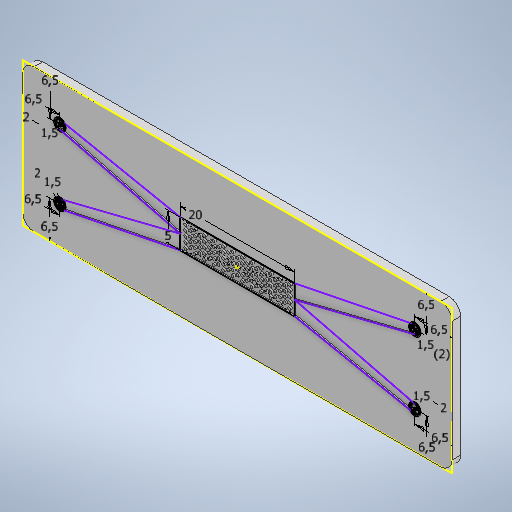
# Autodesk Inventor part: LAB1
Saved by Autodesk Inventor 2025.1 (Build 291241020, 241B)
## iProperties
Created: 2024-09-21
Part Number: LAB1
Material: Generic
Document SubType Name: Modeling
Designer: tomky
Density: 1 g/cm^3
Appearance: Default
Author: tomky
Autodesk Inventor part; units mm, degrees
ref_plane "YZ Plane" through (0, 0, 0) normal (1, 0, 0) x (0, 1, 0)
ref_plane "XZ Plane" through (0, 0, 0) normal (0, 1, 0) x (-1, 0, 0)
ref_plane "XY Plane" through (0, 0, 0) normal (0, 0, 1) x (1, 0, 0)
sketch "Sketch1" plane through (0, 0, 0) normal (0, 0, 1) x (1, 0, 0)
  line L0 (-37.5, 12.5) -> (37.5, 12.5)
  line L1 (37.5, 12.5) -> (37.5, -12.5)
  line L2 (37.5, -12.5) -> (-37.5, -12.5)
  line L3 (-37.5, -12.5) -> (-37.5, 12.5)
  line L4 (-37.5, 12.5) -> (37.5, -12.5) construction
  line L5 (37.5, 12.5) -> (-37.5, -12.5) construction
  point P0 (0, 0)
  dimension "d0" = 75
  dimension "d1" = 25
  constraints: 12 end point, 2 midpoint, 2 parallel, 1 horizontal, 1 perpendicular
  measures "d0" distance of L0.start L0.end
  measures "d1" distance of L0.end L1.end
extrude "Extrusion1" add sketch "Sketch1" along normal blind 1.5
sketch "Sketch2" plane through (0, 0, 1.5) normal (0, 0, 1) x (1, 0, 0)
  line L0 (-37.5, -12.5) -> (37.5, -12.5) projected
  circle A0 centre (31, -6) radius 1
  line L1 (37.5, -12.5) -> (37.5, 12.5) projected
  circle A1 centre (31, 6) radius 1
  line L2 (37.5, 12.5) -> (-37.5, 12.5) projected
  circle A2 centre (-31, 6) radius 1
  line L3 (-37.5, 12.5) -> (-37.5, -12.5) projected
  circle A3 centre (-31, -6) radius 1
  circle A4 centre (-31, 6) radius 0.75
  circle A5 centre (-31, -6) radius 0.75
  circle A6 centre (31, -6) radius 0.75
  circle A7 centre (31, 6) radius 0.75
  line L4 (10, -2.5) -> (-10, -2.5)
  line L5 (-10, -2.5) -> (-10, 2.5)
  line L6 (-10, 2.5) -> (10, 2.5)
  line L7 (10, 2.5) -> (10, -2.5)
  line L8 (10, -2.5) -> (-10, 2.5) construction
  line L9 (-10, -2.5) -> (10, 2.5) construction
  line L10 (31, 6.75) -> (10, 2.5)
  line L11 (31, 5.25) -> (10, 0)
  line L12 (31, -5.25) -> (10, 0)
  line L13 (31, -6.75) -> (10, -2.5)
  line L14 (-31, -5.25) -> (-10, 0)
  line L15 (-31, -6.75) -> (-10, -2.5)
  line L16 (-31, 5.25) -> (-10, 0)
  line L17 (-31, 6.75) -> (-10, 2.5)
  point P0 (0, 0)
  point P1 (30.1897, 6.586)
  point P2 (-30.1897, 6.586)
  point P3 (-30.511, 5.1277)
  point P4 (-30.511, -5.1277)
  point P5 (-30.1897, -6.586)
  point P6 (30.1897, -6.586)
  point P7 (30.511, -5.1277)
  point P8 (30.511, 5.1277)
  dimension "d6" = 2
  dimension "d7" = 6.5
  dimension "d8" = 6.5
  dimension "d9" = 2
  dimension "d10" = 6.5
  dimension "d11" = 6.5
  dimension "d12" = 2
  dimension "d13" = 6.5
  dimension "d14" = 6.5
  dimension "d15" = 2
  dimension "d16" = 6.5
  dimension "d17" = 6.5
  dimension "d18" = 1.5
  dimension "d19" = 1.5
  dimension "d20" = 1.5
  dimension "d21" = 1.5
  dimension "d22" = 20
  dimension "d23" = 5
  constraints: 28 end point, 8 centre point, 8 point on circle, 4 coincident, 4 midpoint, 3 parallel, 1 equal radius, 1 horizontal, 1 perpendicular
  measures "d6" diameter of A0
  measures "d7" distance from line of L0 A0.centre
  measures "d8" distance from line of L1 A0.centre
  measures "d9" diameter of A1
  measures "d10" distance from line of L1 A1.centre
  measures "d11" distance from line of L2 A1.centre
  measures "d12" diameter of A2
  measures "d13" distance from line of L2 A2.centre
  measures "d14" distance from line of L3 A2.centre
  measures "d15" diameter of A3
  measures "d16" distance from line of L3 A3.centre
  measures "d17" distance from line of L0 A3.centre
  measures "d18" diameter of A4
  measures "d19" diameter of A5
  measures "d20" diameter of A6
  measures "d21" diameter of A7
  measures "d22" distance of L5.end L6.end
  measures "d23" distance of L4.end L5.end
extrude "Extrusion2" add sketch "Sketch2" against normal blind 6.5 contours A0 L13 A6 L12 | L12 A6 L13 A0 | A6 L13 | L13 A6 | L11 A7 L10 A1 | A1 L10 A7 L11 | A7 L10 | L15 A5 L14 A3 | A3 L14 A5 L15 | L17 A4 L16 A2 | A2 L16 A4 L17 | A7 L10 | L15 A5 | A5 L15 | L17 A4 | A4 L17
extrude "Extrusion3" cut sketch "Sketch2" against normal through all contours A6 L13 | L13 A6 | A7 L10 | A7 L10 | L15 A5 | A5 L15 | L17 A4 | A4 L17
fillet "Fillet1" radius 0.5 4 edges at (30, 6, 0) (30, -6, 0) (-32, -6, 0) (-32, 6, 0)
extrude "Extrusion4" cut sketch "Sketch2" against normal blind 0.3 contours A0 L13 A6 L12 | L12 A6 L13 A0 | A0 L13 L7 L12 | A6 L13 | L7 L4 L5 L6 | L7 L10 A1 L11 | L13 A6 | L11 A7 L10 A1 | A1 L10 A7 L11 | L15 A3 L14 L5 | L5 L16 A2 L17 | A7 L10 | L15 A5 L14 A3 | A3 L14 A5 L15 | L17 A4 L16 A2 | A2 L16 A4 L17 | A7 L10 | L15 A5 | A5 L15 | L17 A4 | A4 L17
sketch "Sketch3" plane through (0, 0, 1.2) normal (0, 0, 1) x (1, 0, 0)
  line L0 (10, -2.5) -> (-10, -2.5) construction
  line L1 (-10, 2.5) -> (10, 2.5) construction
  line L2 (0, 2.5) -> (0, -2.5) construction
  line L3 (-30.511, -5.1277) -> (-10, 0) projected
  line L4 (30.511, 5.1277) -> (10, 0) projected
  line L5 (-10, 0) -> (10, 0) construction
  circle A0 centre (0, 0.4) radius 0.25
  circle A1 centre (0, 1.3) radius 0.25
  circle A2 centre (0.8062, 0) radius 0.25
  circle A3 centre (0.8062, 0.9) radius 0.25
  circle A4 centre (0.8062, 1.8) radius 0.25
  circle A5 centre (2.4562, 0) radius 0.25
  circle A6 centre (2.4562, 0.9) radius 0.25
  circle A7 centre (2.4562, 1.8) radius 0.25
  circle A8 centre (1.65, 0.4) radius 0.25
  circle A9 centre (1.65, 1.3) radius 0.25
  circle A10 centre (4.1062, 0) radius 0.25
  circle A11 centre (4.1062, 0.9) radius 0.25
  circle A12 centre (4.1062, 1.8) radius 0.25
  circle A13 centre (3.3, 0.4) radius 0.25
  circle A14 centre (3.3, 1.3) radius 0.25
  circle A15 centre (5.7562, 0) radius 0.25
  circle A16 centre (5.7562, 0.9) radius 0.25
  circle A17 centre (5.7562, 1.8) radius 0.25
  circle A18 centre (4.95, 0.4) radius 0.25
  circle A19 centre (4.95, 1.3) radius 0.25
  circle A20 centre (7.4062, 0) radius 0.25
  circle A21 centre (7.4062, 0.9) radius 0.25
  circle A22 centre (7.4062, 1.8) radius 0.25
  circle A23 centre (6.6, 0.4) radius 0.25
  circle A24 centre (6.6, 1.3) radius 0.25
  circle A25 centre (9.0562, 0) radius 0.25
  circle A26 centre (9.0562, 0.9) radius 0.25
  circle A27 centre (9.0562, 1.8) radius 0.25
  circle A28 centre (8.25, 0.4) radius 0.25
  circle A29 centre (8.25, 1.3) radius 0.25
  circle A30 centre (10.7062, 0) radius 0.25
  circle A31 centre (10.7062, 0.9) radius 0.25
  circle A32 centre (10.7062, 1.8) radius 0.25
  circle A33 centre (9.9, 0.4) radius 0.25
  circle A34 centre (9.9, 1.3) radius 0.25
  circle A35 centre (-1.65, 1.3) radius 0.25
  circle A36 centre (-1.65, 0.4) radius 0.25
  circle A37 centre (-0.8438, 0) radius 0.25
  circle A38 centre (-0.8438, 0.9) radius 0.25
  circle A39 centre (-0.8438, 1.8) radius 0.25
  circle A40 centre (-3.3, 1.3) radius 0.25
  circle A41 centre (-3.3, 0.4) radius 0.25
  circle A42 centre (-2.4938, 0) radius 0.25
  circle A43 centre (-2.4938, 0.9) radius 0.25
  circle A44 centre (-2.4938, 1.8) radius 0.25
  circle A45 centre (-4.95, 1.3) radius 0.25
  circle A46 centre (-4.95, 0.4) radius 0.25
  circle A47 centre (-4.1438, 0) radius 0.25
  circle A48 centre (-4.1438, 0.9) radius 0.25
  circle A49 centre (-4.1438, 1.8) radius 0.25
  circle A50 centre (-6.6, 1.3) radius 0.25
  circle A51 centre (-6.6, 0.4) radius 0.25
  circle A52 centre (-5.7938, 0) radius 0.25
  circle A53 centre (-5.7938, 0.9) radius 0.25
  circle A54 centre (-5.7938, 1.8) radius 0.25
  circle A55 centre (-8.25, 1.3) radius 0.25
  circle A56 centre (-8.25, 0.4) radius 0.25
  circle A57 centre (-7.4438, 0) radius 0.25
  circle A58 centre (-7.4438, 0.9) radius 0.25
  circle A59 centre (-7.4438, 1.8) radius 0.25
  circle A60 centre (-9.9, 1.3) radius 0.25
  circle A61 centre (-9.9, 0.4) radius 0.25
  circle A62 centre (-9.0938, 0) radius 0.25
  circle A63 centre (-9.0938, 0.9) radius 0.25
  circle A64 centre (-9.0938, 1.8) radius 0.25
  line L6 (-10, -2.5) -> (10, -2.5) construction
  circle A65 centre (0, -0.4) radius 0.25
  circle A66 centre (0, -1.3) radius 0.25
  circle A67 centre (0.8062, 0) radius 0.25
  circle A68 centre (0.8062, -0.9) radius 0.25
  circle A69 centre (0.8062, -1.8) radius 0.25
  circle A70 centre (2.4562, 0) radius 0.25
  circle A71 centre (2.4562, -0.9) radius 0.25
  circle A72 centre (2.4562, -1.8) radius 0.25
  circle A73 centre (1.65, -0.4) radius 0.25
  circle A74 centre (1.65, -1.3) radius 0.25
  circle A75 centre (4.1062, 0) radius 0.25
  circle A76 centre (4.1062, -0.9) radius 0.25
  circle A77 centre (4.1062, -1.8) radius 0.25
  circle A78 centre (3.3, -0.4) radius 0.25
  circle A79 centre (3.3, -1.3) radius 0.25
  circle A80 centre (5.7562, 0) radius 0.25
  circle A81 centre (5.7562, -0.9) radius 0.25
  circle A82 centre (5.7562, -1.8) radius 0.25
  circle A83 centre (4.95, -0.4) radius 0.25
  circle A84 centre (4.95, -1.3) radius 0.25
  circle A85 centre (7.4062, 0) radius 0.25
  circle A86 centre (7.4062, -0.9) radius 0.25
  circle A87 centre (7.4062, -1.8) radius 0.25
  circle A88 centre (6.6, -0.4) radius 0.25
  circle A89 centre (6.6, -1.3) radius 0.25
  circle A90 centre (9.0562, 0) radius 0.25
  circle A91 centre (9.0562, -0.9) radius 0.25
  circle A92 centre (9.0562, -1.8) radius 0.25
  circle A93 centre (8.25, -0.4) radius 0.25
  circle A94 centre (8.25, -1.3) radius 0.25
  circle A95 centre (9.9, -0.4) radius 0.25
  circle A96 centre (9.9, -1.3) radius 0.25
  circle A97 centre (-1.65, -1.3) radius 0.25
  circle A98 centre (-1.65, -0.4) radius 0.25
  circle A99 centre (-0.8438, 0) radius 0.25
  circle A100 centre (-0.8438, -0.9) radius 0.25
  circle A101 centre (-0.8438, -1.8) radius 0.25
  circle A102 centre (-3.3, -1.3) radius 0.25
  circle A103 centre (-3.3, -0.4) radius 0.25
  circle A104 centre (-2.4938, 0) radius 0.25
  circle A105 centre (-2.4938, -0.9) radius 0.25
  circle A106 centre (-2.4938, -1.8) radius 0.25
  circle A107 centre (-4.95, -1.3) radius 0.25
  circle A108 centre (-4.95, -0.4) radius 0.25
  circle A109 centre (-4.1438, 0) radius 0.25
  circle A110 centre (-4.1438, -0.9) radius 0.25
  circle A111 centre (-4.1438, -1.8) radius 0.25
  circle A112 centre (-6.6, -1.3) radius 0.25
  circle A113 centre (-6.6, -0.4) radius 0.25
  circle A114 centre (-5.7938, 0) radius 0.25
  circle A115 centre (-5.7938, -0.9) radius 0.25
  circle A116 centre (-5.7938, -1.8) radius 0.25
  circle A117 centre (-8.25, -1.3) radius 0.25
  circle A118 centre (-8.25, -0.4) radius 0.25
  circle A119 centre (-7.4438, 0) radius 0.25
  circle A120 centre (-7.4438, -0.9) radius 0.25
  circle A121 centre (-7.4438, -1.8) radius 0.25
  circle A122 centre (-9.9, -1.3) radius 0.25
  circle A123 centre (-9.9, -0.4) radius 0.25
  circle A124 centre (-9.0938, 0) radius 0.25
  circle A125 centre (-9.0938, -0.9) radius 0.25
  circle A126 centre (-9.0938, -1.8) radius 0.25
  point P0 (0, 0)
  point P1 (0, 0)
  point P2 (1.65, 0)
  point P3 (3.3, 0)
  point P4 (4.95, 0)
  point P5 (6.6, 0)
  point P6 (8.25, 0)
  point P7 (9.9, 0)
  point P8 (-1.65, 0)
  point P9 (-1.65, 0)
  point P10 (-3.3, 0)
  point P11 (-3.3, 0)
  point P12 (-4.95, 0)
  point P13 (-4.95, 0)
  point P14 (-6.6, 0)
  point P15 (-6.6, 0)
  point P16 (-8.25, 0)
  point P17 (-8.25, 0)
  point P18 (-9.9, 0)
  point P19 (-9.9, 0)
  dimension "d31" = 0.5
  dimension "d32" = 0
  dimension "d33" = 0.4
  dimension "d34" = 0.5
  dimension "d35" = 0.4
  dimension "d36" = 0.5
  dimension "d37" = 0.4
  dimension "d38" = 0.5
  dimension "d41" = 0.4
  dimension "d42" = 0.5
  dimension "d43" = 0.4
  dimension "d46" = 1.65
  dimension "d53" = 1.65
  constraints: 127 centre point, 50 symmetric about line, 6 end point, 3 midpoint, 2 horizontal, 2 point on line, 2 vertical alignment, 1 perpendicular, 200 other
  measures "d31" diameter of A0
  measures "d32" distance from line of L2 A0.centre
  measures "d33" distance of point (0, 0) A0.centre
  measures "d34" diameter of A1
  measures "d36" diameter of A2
  measures "d37" vertical distance between centres of A0 A2
  measures "d38" diameter of A3
  measures "d42" diameter of A4
  measures "d46" distance of A0.centre A8.centre
  measures "d53" distance of A1.centre A35.centre
extrude "Extrusion5" add sketch "Sketch3" along normal blind 0.3 contours A0 | A1 | A2 | A3 | A4 | A5 | A6 | A7 | A8 | A9 | A10 | A11 | A12 | A13 | A14 | A15 | A16 | A17 | A18 | A19 | A20 | A21 | A22 | A23 | A24 | A25 | A26 | A27 | A28 | A29 | A35 | A36 | A37 | A38 | A39 | A40 | A41 | A42 | A43 | A44 | A45 | A46 | A47 | A48 | A49 | A50 | A51 | A52 | A53 | A54 | A55 | A56 | A57 | A58 | A59 | A62 | A63 | A64 | A65 | A66 | A68 | A69 | A71 | A72 | A73 | A74 | A76 | A77 | A78 | A79 | A81 | A82 | A83 | A84 | A86 | A87 | A88 | A89 | A91 | A92 | A93 | A94 | A97 | A98 | A100 | A101 | A102 | A103 | A105 | A106 | A107 | A108 | A110 | A111 | A112 | A113 | A115 | A116 | A117 | A118 | A120 | A121 | A125 | A126
sketch "Sketch4" plane through (0, 0, 0) normal (0, 0, -1) x (-1, 0, 0)
  line L0 (35.8622, -11.4875) -> (8.2993, -11.4875) construction
  line L1 (8.2993, -11.4875) -> (8.2993, -8.311) construction
  line L2 (8.2993, -8.311) -> (35.8622, -8.311) construction
  line L3 (35.8622, -8.311) -> (35.8622, -11.4875) construction
  line L4 (35.0121, -8.894) -> (35.0121, -11.1335)
  line L5 (35.0121, -11.1335) -> (35.8643, -11.1335)
  line L6 (35.8643, -11.1335) -> (35.8643, -11.434)
  line L7 (35.8643, -11.434) -> (33.8224, -11.434)
  line L8 (33.8224, -11.434) -> (33.8224, -11.1335)
  line L9 (33.8224, -11.1335) -> (34.6745, -11.1335)
  line L10 (34.6745, -11.1335) -> (34.6745, -8.894)
  line L11 (34.6745, -8.894) -> (35.0121, -8.894)
  line L12 (31.7126, -8.894) -> (32.151, -8.894)
  line L13 (32.151, -8.894) -> (33.0793, -10.0755)
  line L14 (33.0793, -10.0755) -> (33.2275, -9.9087)
  line L15 (33.2275, -9.9087) -> (33.2275, -8.894)
  line L16 (33.2275, -8.894) -> (33.5651, -8.894)
  line L17 (33.5651, -8.894) -> (33.5651, -11.434)
  line L18 (33.5651, -11.434) -> (33.2275, -11.434)
  line L19 (33.2275, -11.434) -> (33.2275, -10.2669)
  line L20 (33.2275, -10.2669) -> (32.186, -11.434)
  line L21 (32.186, -11.434) -> (31.7743, -11.434)
  line L22 (31.7743, -11.434) -> (32.8261, -10.2998)
  line L23 (32.8261, -10.2998) -> (31.7126, -8.894)
  line L24 (28.9256, -8.894) -> (30.492, -8.894)
  line L25 (30.492, -8.894) -> (30.492, -9.2542)
  spline S0 degree 2 poles (30.492, -9.2542) (30.3232, -9.4127) (30.0227, -9.707) (29.8786, -9.8655) knots 0 0 0 1 2 2 2
  spline S1 degree 2 poles (29.8786, -9.8655) (29.5884, -10.1846) (29.3764, -10.5674) (29.3764, -10.7712) knots 0 0 0 1 2 2 2
  spline S2 degree 2 poles (29.3764, -10.7712) (29.3764, -10.8782) (29.4422, -11.0388) (29.5019, -11.0902) knots 0 0 0 1 2 2 2
  spline S3 degree 2 poles (29.5019, -11.0902) (29.5616, -11.1417) (29.718, -11.1931) (29.8127, -11.1931) knots 0 0 0 1 2 2 2
  spline S4 degree 2 poles (29.8127, -11.1931) (29.9033, -11.1931) (30.0885, -11.1479) (30.1729, -11.1129) knots 0 0 0 1 2 2 2
  spline S5 degree 2 poles (30.1729, -11.1129) (30.245, -11.0841) (30.3788, -11.0017) (30.4199, -10.9729) knots 0 0 0 1 2 2 2
  line L26 (30.4199, -10.9729) -> (30.4385, -10.9729)
  line L27 (30.4385, -10.9729) -> (30.4385, -11.3352)
  spline S6 degree 2 poles (30.4385, -11.3352) (30.3335, -11.3866) (29.9568, -11.4875) (29.788, -11.4875) knots 0 0 0 1 2 2 2
  spline S7 degree 2 poles (29.788, -11.4875) (29.4319, -11.4875) (29.0306, -11.1108) (29.0306, -10.7897) knots 0 0 0 1 2 2 2
  spline S8 degree 2 poles (29.0306, -10.7897) (29.0306, -10.6395) (29.1005, -10.3883) (29.1623, -10.2813) knots 0 0 0 1 2 2 2
  spline S9 degree 2 poles (29.1623, -10.2813) (29.224, -10.1701) (29.4031, -9.952) (29.5019, -9.847) knots 0 0 0 1 2 2 2
  spline S10 degree 2 poles (29.5019, -9.847) (29.6625, -9.672) (30.0556, -9.2974) (30.1729, -9.1883) knots 0 0 0 1 2 2 2
  line L28 (30.1729, -9.1883) -> (28.9256, -9.1883)
  line L29 (28.9256, -9.1883) -> (28.9256, -8.894)
  line L30 (27.0195, -8.894) -> (28.586, -8.894)
  line L31 (28.586, -8.894) -> (28.586, -9.2542)
  spline S11 degree 2 poles (28.586, -9.2542) (28.4172, -9.4127) (28.1166, -9.707) (27.9726, -9.8655) knots 0 0 0 1 2 2 2
  spline S12 degree 2 poles (27.9726, -9.8655) (27.6823, -10.1846) (27.4703, -10.5674) (27.4703, -10.7712) knots 0 0 0 1 2 2 2
  spline S13 degree 2 poles (27.4703, -10.7712) (27.4703, -10.8782) (27.5362, -11.0388) (27.5959, -11.0902) knots 0 0 0 1 2 2 2
  spline S14 degree 2 poles (27.5959, -11.0902) (27.6556, -11.1417) (27.812, -11.1931) (27.9067, -11.1931) knots 0 0 0 1 2 2 2
  spline S15 degree 2 poles (27.9067, -11.1931) (27.9973, -11.1931) (28.1825, -11.1479) (28.2669, -11.1129) knots 0 0 0 1 2 2 2
  spline S16 degree 2 poles (28.2669, -11.1129) (28.3389, -11.0841) (28.4727, -11.0017) (28.5139, -10.9729) knots 0 0 0 1 2 2 2
  line L32 (28.5139, -10.9729) -> (28.5324, -10.9729)
  line L33 (28.5324, -10.9729) -> (28.5324, -11.3352)
  spline S17 degree 2 poles (28.5324, -11.3352) (28.4275, -11.3866) (28.0508, -11.4875) (27.882, -11.4875) knots 0 0 0 1 2 2 2
  spline S18 degree 2 poles (27.882, -11.4875) (27.5259, -11.4875) (27.1245, -11.1108) (27.1245, -10.7897) knots 0 0 0 1 2 2 2
  spline S19 degree 2 poles (27.1245, -10.7897) (27.1245, -10.6395) (27.1945, -10.3883) (27.2563, -10.2813) knots 0 0 0 1 2 2 2
  spline S20 degree 2 poles (27.2563, -10.2813) (27.318, -10.1701) (27.4971, -9.952) (27.5959, -9.847) knots 0 0 0 1 2 2 2
  spline S21 degree 2 poles (27.5959, -9.847) (27.7564, -9.672) (28.1496, -9.2974) (28.2669, -9.1883) knots 0 0 0 1 2 2 2
  line L34 (28.2669, -9.1883) -> (27.0195, -9.1883)
  line L35 (27.0195, -9.1883) -> (27.0195, -8.894)
  line L36 (25.7495, -9.8511) -> (26.7108, -9.8511)
  line L37 (26.7108, -9.8511) -> (26.7108, -10.1599)
  line L38 (26.7108, -10.1599) -> (25.7495, -10.1599)
  line L39 (25.7495, -10.1599) -> (25.7495, -9.8511)
  spline S22 degree 2 poles (23.8312, -10.164) (23.8312, -9.4806) (24.2284, -8.8405) (24.6422, -8.8405) knots 0 0 0 1 2 2 2
  spline S23 degree 2 poles (24.6422, -8.8405) (25.0621, -8.8405) (25.4552, -9.493) (25.4552, -10.1619) knots 0 0 0 1 2 2 2
  spline S24 degree 2 poles (25.4552, -10.1619) (25.4552, -10.8494) (25.0579, -11.4854) (24.6422, -11.4854) knots 0 0 0 1 2 2 2
  spline S25 degree 2 poles (24.6422, -11.4854) (24.2243, -11.4854) (23.8312, -10.8268) (23.8312, -10.164) knots 0 0 0 1 2 2 2
  spline S26 degree 2 poles (24.2675, -9.39) (24.2181, -9.5156) (24.177, -9.9026) (24.177, -10.164) knots 0 0 0 1 2 2 2
  spline S27 degree 2 poles (24.177, -10.164) (24.177, -10.4254) (24.2181, -10.8103) (24.2696, -10.94) knots 0 0 0 1 2 2 2
  spline S28 degree 2 poles (24.2696, -10.94) (24.3211, -11.0696) (24.5001, -11.2034) (24.6422, -11.2034) knots 0 0 0 1 2 2 2
  spline S29 degree 2 poles (24.6422, -11.2034) (24.7842, -11.2034) (24.9674, -11.0696) (25.0209, -10.9359) knots 0 0 0 1 2 2 2
  spline S30 degree 2 poles (25.0209, -10.9359) (25.0724, -10.8062) (25.1094, -10.411) (25.1094, -10.1619) knots 0 0 0 1 2 2 2
  spline S31 degree 2 poles (25.1094, -10.1619) (25.1094, -9.8943) (25.0765, -9.5362) (25.023, -9.3962) knots 0 0 0 1 2 2 2
  spline S32 degree 2 poles (25.023, -9.3962) (24.9736, -9.2645) (24.7904, -9.1224) (24.6422, -9.1224) knots 0 0 0 1 2 2 2
  spline S33 degree 2 poles (24.6422, -9.1224) (24.5022, -9.1224) (24.319, -9.2562) (24.2675, -9.39) knots 0 0 0 1 2 2 2
  spline S34 degree 2 poles (23.5759, -10.6086) (23.5759, -10.8041) (23.4483, -11.1293) (23.3372, -11.2467) knots 0 0 0 1 2 2 2
  spline S35 degree 2 poles (23.3372, -11.2467) (23.2322, -11.3599) (22.9255, -11.4854) (22.7691, -11.4854) knots 0 0 0 1 2 2 2
  spline S36 degree 2 poles (22.7691, -11.4854) (22.5941, -11.4854) (22.3101, -11.3681) (22.2051, -11.257) knots 0 0 0 1 2 2 2
  spline S37 degree 2 poles (22.2051, -11.257) (22.0733, -11.117) (21.9293, -10.6642) (21.9293, -10.3163) knots 0 0 0 1 2 2 2
  spline S38 degree 2 poles (21.9293, -10.3163) (21.9293, -10.0014) (22.0713, -9.4374) (22.2092, -9.2501) knots 0 0 0 1 2 2 2
  spline S39 degree 2 poles (22.2092, -9.2501) (22.3553, -9.0525) (22.767, -8.8446) (23.0675, -8.8446) knots 0 0 0 1 2 2 2
  spline S40 degree 2 poles (23.0675, -8.8446) (23.1354, -8.8446) (23.2898, -8.859) (23.3557, -8.8796) knots 0 0 0 1 2 2 2
  line L40 (23.3557, -8.8796) -> (23.3557, -9.2068)
  line L41 (23.3557, -9.2068) -> (23.3392, -9.2068)
  spline S41 degree 2 poles (23.3392, -9.2068) (23.296, -9.1821) (23.1149, -9.1389) (23.0222, -9.1389) knots 0 0 0 1 2 2 2
  spline S42 degree 2 poles (23.0222, -9.1389) (22.6888, -9.1389) (22.308, -9.5794) (22.2812, -9.987) knots 0 0 0 1 2 2 2
  spline S43 degree 2 poles (22.2812, -9.987) (22.4171, -9.8943) (22.6641, -9.8099) (22.8102, -9.8099) knots 0 0 0 1 2 2 2
  spline S44 degree 2 poles (22.8102, -9.8099) (22.9502, -9.8099) (23.1828, -9.8717) (23.3001, -9.9602) knots 0 0 0 1 2 2 2
  spline S45 degree 2 poles (23.3001, -9.9602) (23.436, -10.0652) (23.5759, -10.3842) (23.5759, -10.6086) knots 0 0 0 1 2 2 2
  spline S46 degree 2 poles (22.273, -10.3924) (22.273, -10.6497) (22.3677, -10.975) (22.4521, -11.0635) knots 0 0 0 1 2 2 2
  spline S47 degree 2 poles (22.4521, -11.0635) (22.5262, -11.1458) (22.6806, -11.2076) (22.7711, -11.2076) knots 0 0 0 1 2 2 2
  spline S48 degree 2 poles (22.7711, -11.2076) (22.9811, -11.2076) (23.2301, -10.907) (23.2301, -10.623) knots 0 0 0 1 2 2 2
  spline S49 degree 2 poles (23.2301, -10.623) (23.2301, -10.4624) (23.1478, -10.2545) (23.0572, -10.1804) knots 0 0 0 1 2 2 2
  spline S50 degree 2 poles (23.0572, -10.1804) (22.9914, -10.1269) (22.8288, -10.0919) (22.7341, -10.0919) knots 0 0 0 1 2 2 2
  spline S51 degree 2 poles (22.7341, -10.0919) (22.625, -10.0919) (22.3739, -10.1681) (22.2792, -10.2319) knots 0 0 0 1 2 2 2
  spline S52 degree 2 poles (22.2792, -10.2319) (22.2771, -10.2566) (22.273, -10.341) (22.273, -10.3924) knots 0 0 0 1 2 2 2
  line L42 (20.6695, -9.8511) -> (21.6308, -9.8511)
  line L43 (21.6308, -9.8511) -> (21.6308, -10.1599)
  line L44 (21.6308, -10.1599) -> (20.6695, -10.1599)
  line L45 (20.6695, -10.1599) -> (20.6695, -9.8511)
  line L46 (18.7656, -8.894) -> (20.332, -8.894)
  line L47 (20.332, -8.894) -> (20.332, -9.2542)
  spline S53 degree 2 poles (20.332, -9.2542) (20.1632, -9.4127) (19.8627, -9.707) (19.7186, -9.8655) knots 0 0 0 1 2 2 2
  spline S54 degree 2 poles (19.7186, -9.8655) (19.4284, -10.1846) (19.2164, -10.5674) (19.2164, -10.7712) knots 0 0 0 1 2 2 2
  spline S55 degree 2 poles (19.2164, -10.7712) (19.2164, -10.8782) (19.2822, -11.0388) (19.3419, -11.0902) knots 0 0 0 1 2 2 2
  spline S56 degree 2 poles (19.3419, -11.0902) (19.4016, -11.1417) (19.558, -11.1931) (19.6527, -11.1931) knots 0 0 0 1 2 2 2
  spline S57 degree 2 poles (19.6527, -11.1931) (19.7433, -11.1931) (19.9285, -11.1479) (20.0129, -11.1129) knots 0 0 0 1 2 2 2
  spline S58 degree 2 poles (20.0129, -11.1129) (20.085, -11.0841) (20.2188, -11.0017) (20.2599, -10.9729) knots 0 0 0 1 2 2 2
  line L48 (20.2599, -10.9729) -> (20.2785, -10.9729)
  line L49 (20.2785, -10.9729) -> (20.2785, -11.3352)
  spline S59 degree 2 poles (20.2785, -11.3352) (20.1735, -11.3866) (19.7968, -11.4875) (19.628, -11.4875) knots 0 0 0 1 2 2 2
  spline S60 degree 2 poles (19.628, -11.4875) (19.2719, -11.4875) (18.8706, -11.1108) (18.8706, -10.7897) knots 0 0 0 1 2 2 2
  spline S61 degree 2 poles (18.8706, -10.7897) (18.8706, -10.6395) (18.9405, -10.3883) (19.0023, -10.2813) knots 0 0 0 1 2 2 2
  spline S62 degree 2 poles (19.0023, -10.2813) (19.064, -10.1701) (19.2431, -9.952) (19.3419, -9.847) knots 0 0 0 1 2 2 2
  spline S63 degree 2 poles (19.3419, -9.847) (19.5025, -9.672) (19.8956, -9.2974) (20.0129, -9.1883) knots 0 0 0 1 2 2 2
  line L50 (20.0129, -9.1883) -> (18.7656, -9.1883)
  line L51 (18.7656, -9.1883) -> (18.7656, -8.894)
  spline S64 degree 2 poles (16.8451, -10.164) (16.8451, -9.4806) (17.2424, -8.8405) (17.6561, -8.8405) knots 0 0 0 1 2 2 2
  spline S65 degree 2 poles (17.6561, -8.8405) (18.076, -8.8405) (18.4692, -9.493) (18.4692, -10.1619) knots 0 0 0 1 2 2 2
  spline S66 degree 2 poles (18.4692, -10.1619) (18.4692, -10.8494) (18.0719, -11.4854) (17.6561, -11.4854) knots 0 0 0 1 2 2 2
  spline S67 degree 2 poles (17.6561, -11.4854) (17.2383, -11.4854) (16.8451, -10.8268) (16.8451, -10.164) knots 0 0 0 1 2 2 2
  spline S68 degree 2 poles (17.2815, -9.39) (17.2321, -9.5156) (17.1909, -9.9026) (17.1909, -10.164) knots 0 0 0 1 2 2 2
  spline S69 degree 2 poles (17.1909, -10.164) (17.1909, -10.4254) (17.2321, -10.8103) (17.2836, -10.94) knots 0 0 0 1 2 2 2
  spline S70 degree 2 poles (17.2836, -10.94) (17.335, -11.0696) (17.5141, -11.2034) (17.6561, -11.2034) knots 0 0 0 1 2 2 2
  spline S71 degree 2 poles (17.6561, -11.2034) (17.7982, -11.2034) (17.9813, -11.0696) (18.0349, -10.9359) knots 0 0 0 1 2 2 2
  spline S72 degree 2 poles (18.0349, -10.9359) (18.0863, -10.8062) (18.1234, -10.411) (18.1234, -10.1619) knots 0 0 0 1 2 2 2
  spline S73 degree 2 poles (18.1234, -10.1619) (18.1234, -9.8943) (18.0904, -9.5362) (18.0369, -9.3962) knots 0 0 0 1 2 2 2
  spline S74 degree 2 poles (18.0369, -9.3962) (17.9875, -9.2645) (17.8043, -9.1224) (17.6561, -9.1224) knots 0 0 0 1 2 2 2
  spline S75 degree 2 poles (17.6561, -9.1224) (17.5162, -9.1224) (17.333, -9.2562) (17.2815, -9.39) knots 0 0 0 1 2 2 2
  line L52 (14.9535, -8.894) -> (16.5199, -8.894)
  line L53 (16.5199, -8.894) -> (16.5199, -9.2542)
  spline S76 degree 2 poles (16.5199, -9.2542) (16.3511, -9.4127) (16.0506, -9.707) (15.9065, -9.8655) knots 0 0 0 1 2 2 2
  spline S77 degree 2 poles (15.9065, -9.8655) (15.6163, -10.1846) (15.4043, -10.5674) (15.4043, -10.7712) knots 0 0 0 1 2 2 2
  spline S78 degree 2 poles (15.4043, -10.7712) (15.4043, -10.8782) (15.4702, -11.0388) (15.5299, -11.0902) knots 0 0 0 1 2 2 2
  spline S79 degree 2 poles (15.5299, -11.0902) (15.5895, -11.1417) (15.746, -11.1931) (15.8407, -11.1931) knots 0 0 0 1 2 2 2
  spline S80 degree 2 poles (15.8407, -11.1931) (15.9312, -11.1931) (16.1165, -11.1479) (16.2009, -11.1129) knots 0 0 0 1 2 2 2
  spline S81 degree 2 poles (16.2009, -11.1129) (16.2729, -11.0841) (16.4067, -11.0017) (16.4479, -10.9729) knots 0 0 0 1 2 2 2
  line L54 (16.4479, -10.9729) -> (16.4664, -10.9729)
  line L55 (16.4664, -10.9729) -> (16.4664, -11.3352)
  spline S82 degree 2 poles (16.4664, -11.3352) (16.3614, -11.3866) (15.9848, -11.4875) (15.816, -11.4875) knots 0 0 0 1 2 2 2
  spline S83 degree 2 poles (15.816, -11.4875) (15.4599, -11.4875) (15.0585, -11.1108) (15.0585, -10.7897) knots 0 0 0 1 2 2 2
  spline S84 degree 2 poles (15.0585, -10.7897) (15.0585, -10.6395) (15.1285, -10.3883) (15.1902, -10.2813) knots 0 0 0 1 2 2 2
  spline S85 degree 2 poles (15.1902, -10.2813) (15.252, -10.1701) (15.4311, -9.952) (15.5299, -9.847) knots 0 0 0 1 2 2 2
  spline S86 degree 2 poles (15.5299, -9.847) (15.6904, -9.672) (16.0836, -9.2974) (16.2009, -9.1883) knots 0 0 0 1 2 2 2
  line L56 (16.2009, -9.1883) -> (14.9535, -9.1883)
  line L57 (14.9535, -9.1883) -> (14.9535, -8.894)
  line L58 (12.9796, -9.7667) -> (13.2821, -9.7667)
  line L59 (13.2821, -9.7667) -> (13.2821, -8.894)
  line L60 (13.2821, -8.894) -> (13.6094, -8.894)
  line L61 (13.6094, -8.894) -> (13.6094, -9.7667)
  line L62 (13.6094, -9.7667) -> (14.7312, -9.7667)
  line L63 (14.7312, -9.7667) -> (14.7312, -10.1249)
  line L64 (14.7312, -10.1249) -> (13.595, -11.434)
  line L65 (13.595, -11.434) -> (13.2821, -11.434)
  line L66 (13.2821, -11.434) -> (13.2821, -10.0405)
  line L67 (13.2821, -10.0405) -> (12.9796, -10.0405)
  line L68 (12.9796, -10.0405) -> (12.9796, -9.7667)
  line L69 (13.6094, -10.0405) -> (13.6094, -11.0326)
  line L70 (13.6094, -11.0326) -> (14.4636, -10.0405)
  line L71 (14.4636, -10.0405) -> (13.6094, -10.0405)
  point P0 (0, 0)
  constraints: 2 other
extrude "Extrusion6" cut sketch "Sketch4" against normal blind 0.5
fillet "Fillet2" radius 2 4 edges at (37.5, -12.5, 0.75) (-37.5, -12.5, 0.75) (-37.5, 12.5, 0.75) (37.5, 12.5, 0.75)
sketch "Sketch5" plane through (-35.5, 12.5, 0) normal (0, 1, 0) x (1, 0, 0)
  circle A0 centre (71.5, -0.75) radius 0.5
  line L0 (71, 0) -> (0, 0) projected
  line L1 (73, -1.5) -> (73, 0) projected
  circle A1 centre (69.5, -0.75) radius 0.5
  circle A2 centre (67.5, -0.75) radius 0.5
  circle A3 centre (65.5, -0.75) radius 0.5
  circle A4 centre (63.5, -0.75) radius 0.5
  circle A5 centre (61.5, -0.75) radius 0.5
  circle A6 centre (59.5, -0.75) radius 0.5
  circle A7 centre (57.5, -0.75) radius 0.5
  circle A8 centre (55.5, -0.75) radius 0.5
  circle A9 centre (53.5, -0.75) radius 0.5
  circle A10 centre (51.5, -0.75) radius 0.5
  circle A11 centre (49.5, -0.75) radius 0.5
  circle A12 centre (47.5, -0.75) radius 0.5
  circle A13 centre (45.5, -0.75) radius 0.5
  circle A14 centre (43.5, -0.75) radius 0.5
  circle A15 centre (41.5, -0.75) radius 0.5
  circle A16 centre (39.5, -0.75) radius 0.5
  circle A17 centre (37.5, -0.75) radius 0.5
  circle A18 centre (35.5, -0.75) radius 0.5
  circle A19 centre (33.5, -0.75) radius 0.5
  circle A20 centre (31.5, -0.75) radius 0.5
  circle A21 centre (29.5, -0.75) radius 0.5
  circle A22 centre (27.5, -0.75) radius 0.5
  circle A23 centre (25.5, -0.75) radius 0.5
  circle A24 centre (23.5, -0.75) radius 0.5
  circle A25 centre (21.5, -0.75) radius 0.5
  circle A26 centre (19.5, -0.75) radius 0.5
  circle A27 centre (17.5, -0.75) radius 0.5
  circle A28 centre (15.5, -0.75) radius 0.5
  circle A29 centre (13.5, -0.75) radius 0.5
  circle A30 centre (11.5, -0.75) radius 0.5
  circle A31 centre (9.5, -0.75) radius 0.5
  circle A32 centre (7.5, -0.75) radius 0.5
  circle A33 centre (5.5, -0.75) radius 0.5
  circle A34 centre (3.5, -0.75) radius 0.5
  circle A35 centre (1.5, -0.75) radius 0.5
  circle A36 centre (-0.5, -0.75) radius 0.5
  point P0 (35.5, 0)
  point P1 (73, -0.75)
  dimension "d63" = 1
  dimension "d64" = 0.75
  dimension "d65" = 1.5
  dimension "d68" = 2
  constraints: 37 centre point, 1 horizontal, 1 midpoint, 72 other
  measures "d63" diameter of A0
  measures "d64" distance from line of L0 A0.centre
  measures "d65" distance of point (73, -0.75) A0.centre
  measures "d68" distance of A0.centre A1.centre
extrude "Extrusion7" [suppressed]
sketch "Sketch6" plane through (18, 22.5, 0.75) normal (0, 1, 0) x (1, 0, 0)
  line L0 (20.5, -1.75) -> (-56.5, -1.75)
  line L1 (-56.5, -1.75) -> (-56.5, 1.75)
  line L2 (-56.5, 1.75) -> (20.5, 1.75)
  line L3 (20.5, 1.75) -> (20.5, -1.75)
  circle A0 centre (-18, 0) radius 0.5 projected
  line L4 (20.5, -1.75) -> (-56.5, 1.75) construction
  line L5 (-56.5, -1.75) -> (20.5, 1.75) construction
  point P0 (-18, 0.75)
  dimension "d75" = 77
  dimension "d76" = 3.5
  constraints: 12 end point, 2 midpoint, 2 parallel, 1 horizontal, 1 perpendicular
  measures "d75" distance of L1.end L2.end
  measures "d76" distance between parallel lines of L0 L2
extrude "Extrusion8" [suppressed]
body "Solid1"
